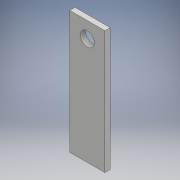
# Autodesk Inventor part: Montant
Saved by Autodesk Inventor 2018 (Build 220112000, 112)
## iProperties
Created: 2018-04-09
Part Number: Montant
Material: Générique
Document SubType Name: Modeling
Designer: Dimitri
Density: 1 g/cm^3
Appearance: Par défaut
Author: Dimitri
Autodesk Inventor part; units mm, degrees
ref_plane "YZ Plane" through (0, 0, 0) normal (1, 0, 0) x (0, 1, 0)
ref_plane "XZ Plane" through (0, 0, 0) normal (0, 1, 0) x (-1, 0, 0)
ref_plane "XY Plane" through (0, 0, 0) normal (0, 0, 1) x (1, 0, 0)
sketch "Esquisse1" plane through (0, 0, 0) normal (0, 1, 0) x (-1, 0, 0)
  line L0 (-10, 35) -> (10, 35)
  line L1 (10, 35) -> (10, -35)
  line L2 (10, -35) -> (-10, -35)
  line L3 (-10, -35) -> (-10, 35)
  line L4 (-10, 35) -> (10, -35) construction
  line L5 (10, 35) -> (-10, -35) construction
  point P0 (0, 0)
  dimension "d0" = 20
  dimension "d1" = 70
  constraints: 12 end point, 2 midpoint, 2 parallel, 1 horizontal, 1 perpendicular
  measures "d0" distance of L1.end L2.end
  measures "d1" distance of L0.end L1.end
extrude "Extrusion1" add sketch "Esquisse1" along normal blind 3
sketch "Esquisse2" plane through (0, 0, 0) normal (0, -1, 0) x (1, 0, 0)
  circle A0 centre (0, 26) radius 4
  line L0 (10, 35) -> (-10, 35) projected
  point P0 (0, 0)
  dimension "d4" = 8
  dimension "d5" = 9
  constraints: 1 centre point
  measures "d4" diameter of A0
  measures "d5" distance from line of L0 A0.centre
extrude "Extrusion2" cut sketch "Esquisse2" against normal blind 3
